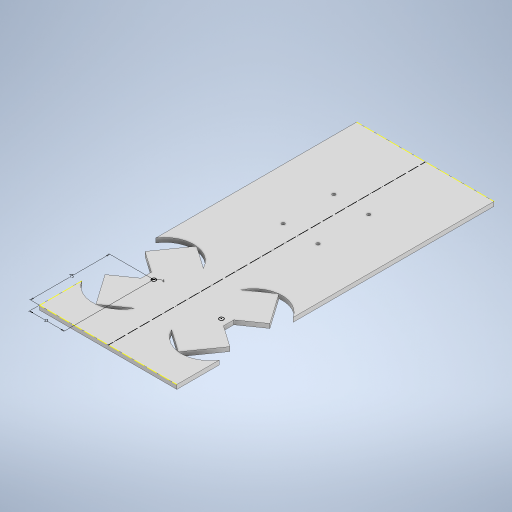
# Autodesk Inventor part: Langbektang houder
Saved by Autodesk Inventor 2023.2 (Build 272271000, 271)
## iProperties
Created: 2020-09-09
Part Number: Langbektang houder
Material: Generic
Document SubType Name: Modeling
Designer: nathan.bollaert
Density: 1 g/cm^3
Appearance: Default
Author: nathan.bollaert
Autodesk Inventor part; units mm, degrees
ref_plane "YZ Plane" through (0, 0, 0) normal (1, 0, 0) x (0, 1, 0)
ref_plane "XZ Plane" through (0, 0, 0) normal (0, 1, 0) x (-1, 0, 0)
ref_plane "XY Plane" through (0, 0, 0) normal (0, 0, 1) x (1, 0, 0)
sketch "Sketch1" plane through (0, 0, 0) normal (0, 1, 0) x (-1, 0, 0)
  line L0 (0, 0) -> (-130, 0)
  line L1 (-130, 0) -> (-130, -300)
  line L2 (-130, -300) -> (0, -300)
  line L3 (0, -40) -> (-26, -40)
  line L4 (-26, -40) -> (-26, -110)
  line L5 (-26, -110) -> (0, -110)
  line L6 (-33, -75) -> (-5.968, -56.072)
  line L7 (-5.968, -56.072) -> (-26.0432, -27.4017)
  line L8 (-26.0432, -27.4017) -> (-47.3411, -42.3146)
  line L9 (-33, -75) -> (-5.968, -93.928)
  line L10 (-5.968, -93.928) -> (-26.0432, -122.5983)
  line L11 (-47.3411, -107.6854) -> (-26.0432, -122.5983)
  arc A0 (0, -40) -> (-47.3411, -42.3146) centre (-23.0242, -54.378) ccw
  arc A1 (-47.3411, -107.6854) -> (0, -110) centre (-23.0242, -95.622) ccw
  line L12 (0, -75) -> (-33, -75)
  line L13 (-33, -75) -> (-26, -75)
  line L14 (-47.3411, -107.6854) -> (-27.4278, -77.1868)
  line L15 (-47.3411, -42.3146) -> (-27.4278, -72.8132)
  arc A2 (-27.4278, -77.1868) -> (-27.4278, -72.8132) centre (-30.7771, -75) ccw
  line L16 (-130, -110) -> (-104, -110)
  line L17 (-104, -110) -> (-104, -40)
  line L18 (-104, -40) -> (-130, -40)
  line L19 (-97, -75) -> (-124.032, -93.928)
  line L20 (-124.032, -93.928) -> (-103.9568, -122.5983)
  line L21 (-103.9568, -122.5983) -> (-82.6589, -107.6854)
  line L22 (-97, -75) -> (-124.032, -56.072)
  line L23 (-124.032, -56.072) -> (-103.9568, -27.4017)
  line L24 (-82.6589, -42.3146) -> (-103.9568, -27.4017)
  arc A3 (-130, -110) -> (-82.6589, -107.6854) centre (-106.9758, -95.622) ccw
  arc A4 (-82.6589, -42.3146) -> (-130, -40) centre (-106.9758, -54.378) ccw
  line L25 (-130, -75) -> (-97, -75)
  line L26 (-97, -75) -> (-104, -75)
  line L27 (-82.6589, -42.3146) -> (-102.5722, -72.8132)
  line L28 (-82.6589, -107.6854) -> (-102.5722, -77.1868)
  arc A5 (-102.5722, -72.8132) -> (-102.5722, -77.1868) centre (-99.2229, -75) ccw
  line L29 (0, -300) -> (0, 0)
  line L30 (0, -260) -> (-26, -260)
  line L31 (-26, -260) -> (-26, -190)
  line L32 (-26, -190) -> (0, -190)
  line L33 (0, -225) -> (-26, -225)
  line L34 (-130, -260) -> (-104, -260)
  line L35 (-104, -260) -> (-104, -190)
  line L36 (-104, -190) -> (-130, -190)
  line L37 (-104, -225) -> (-130, -225)
  point P0 (-101.8038, -71.6364)
  point P1 (-104, -70.0985)
  point P2 (-104, -79.9015)
  point P3 (-101.8038, -78.3636)
  point P4 (-28.1962, -78.3636)
  point P5 (-26, -79.9015)
  point P6 (-26, -70.0985)
  point P7 (-28.1962, -71.6364)
  point P8 (-17.2217, -40)
  point P9 (-17.2217, -110)
  point P10 (-112.7783, -40)
  point P11 (-112.7783, -110)
  dimension "d122" = 130
  dimension "d123" = 300
  dimension "d128" = 75
  dimension "d158" = 33
  dimension "d159" = 35
  dimension "d160" = 35
  dimension "d161" = 4
  dimension "d169" = 35
  dimension "d170" = 35
  dimension "d172" = 75
  dimension "d175" = 33
  dimension "d179" = 33
  dimension "d183" = 70
  dimension "d185" = 26
  dimension "d186" = 35
  dimension "d187" = 26
  dimension "d188" = 75
  dimension "d189" = 70
  dimension "d190" = 26
  dimension "d191" = 75
  constraints: 76 end point, 18 perpendicular, 17 point on line, 16 equal length, 16 point on circle, 6 centre point, 4 horizontal, 4 midpoint, 4 tangent, 3 parallel, 2 coincident, 1 equal radius, 1 vertical, 3 other
  measures "d122" distance of L2.end L1.end
  measures "d123" distance of L1.end L0.end
  measures "d128" distance of L0.start L12.start
  measures "d158" distance of L12.start L12.end
  measures "d159" angle of L12 L6
  measures "d160" angle of L9 L12
  measures "d161" radius of A2
  measures "d169" angle of L25 L19
  measures "d170" angle of L22 L25
  measures "d172" vertical distance of L0.end L25.end
  measures "d175" distance of L6.start L6.end
  measures "d179" distance from line of L23 L25.end
  measures "d183" distance between parallel lines of L18 L16
  measures "d185" distance of L20.end L21.end
  measures "d186" distance of L20.start L20.end
  measures "d187" distance of L17.end L18.end
  measures "d188" distance of L2.end L33.start
  measures "d189" distance of L30.end L31.end
  measures "d190" distance of L30.start L30.end
  measures "d191" distance of L1.end L37.end
extrude "Extrusion1" add sketch "Sketch1" along normal blind 4 contours L29 A0 L15 L6 L9 L14 A1 L32 L31 L30 L2 L1 L34 L35 L36 A3 L28 L19 L22 L27 A4 L0 | L7 L6 L4 L3 | L3 L4 L6 L15 L8 L7 | L23 L24 L27 L22 L17 L18 | L18 L17 L22 L23 | L12 A2 L15 L6 L4 | L4 L9 L14 A2 L12 | L25 A5 L28 L19 L17 | L17 L22 L27 A5 L25 | L15 A2 L12 L6 | L9 L10 L5 L4 | L4 L5 L10 L11 L14 L9 | A2 L14 L9 L12 | L29 L33 L31 L32 | L36 L35 L37 L1 | L20 L19 L17 L16 | L16 L17 L19 L28 L21 L20 | A5 L27 L22 L25 | L25 L19 L28 A5 | L29 L30 L31 L33 | L37 L35 L34 L1
sketch "Sketch12" plane through (0, 4, 0) normal (0, 1, 0) x (1, 0, 0)
  circle A0 centre (48.5, 182) radius 1.5
  circle A1 centre (48.5, 230) radius 1.5
  circle A2 centre (81.5, 230) radius 1.5
  circle A3 centre (81.5, 182) radius 1.5
  line L0 (130, 300) -> (0, 300) projected
  line L1 (0, 300) -> (0, 110) projected
  line L2 (0, 225) -> (130, 225)
  line L3 (130, 110) -> (130, 300) projected
  line L4 (0, 223.5) -> (130, 223.5)
  line L5 (130, 226.5) -> (0, 226.5)
  line L6 (0, 0) -> (130, 0) projected
  line L7 (65, 0) -> (65, 300)
  point P0 (0, 225)
  point P1 (0, 190)
  point P2 (130, 190)
  dimension "d196" = 3
  dimension "d201" = 33
  dimension "d202" = 48
  dimension "d205" = 75
  dimension "d208" = 3
  dimension "d209" = 5
  constraints: 6 end point, 4 centre point, 3 equal radius, 2 horizontal, 2 horizontal alignment, 2 midpoint, 2 point on line, 2 vertical alignment, 1 parallel, 1 symmetric about line, 3 other
  measures "d196" diameter of A0
  measures "d201" distance of A3.centre A0.centre
  measures "d202" distance of A0.centre A1.centre
  measures "d208" distance between parallel lines of L5 L4
hole "Hole1" at (48.5, 4, -182) at (48.5, 4, -230) at (81.5, 4, -182) at (81.5, 4, -230) direction (0, -1, 0) diameter 3 end through all
sketch "Sketch13" plane through (0, 4, 0) normal (0, 1, 0) x (1, 0, 0)
  circle A0 centre (33, 75) radius 2
  line L0 (0, 0) -> (130, 0) projected
  line L1 (0, 40) -> (0, 0) projected
  circle A1 centre (33, 75) radius 2 projected
  line L2 (65, 0) -> (65, 300)
  line L3 (130, 300) -> (0, 300) projected
  circle A2 centre (97, 75) radius 2
  dimension "d217" = 75
  dimension "d219" = 4
  dimension "d220" = 33
  constraints: 2 centre point, 2 end point, 2 midpoint, 1 other
  measures "d217" distance from line of L0 A0.centre
  measures "d219" diameter of A0
  measures "d220" distance from line of L1 A0.centre
body "Solid4"
